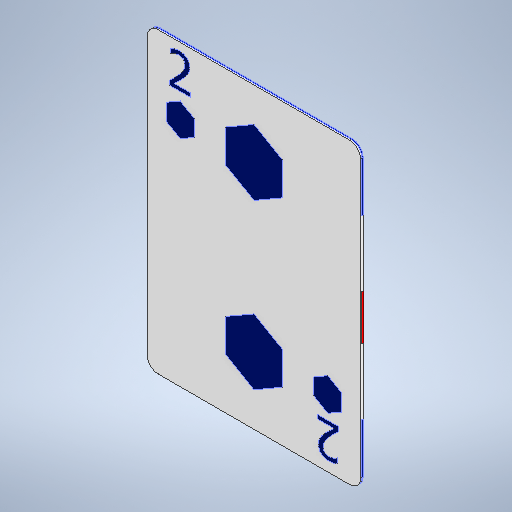
# Autodesk Inventor part: 2ofhexagons
Saved by Autodesk Inventor 2025 (Build 290162010, 162A)
## iProperties
Created: 2024-07-12
Part Number: 2ofhexagons
Material: Generic
Document SubType Name: Modeling
Designer: joshu
Density: 1 g/cm^3
Appearance: Default
Author: joshu
Autodesk Inventor part; units mm, degrees
(part 1 of 3)
ref_plane "YZ Plane" through (0, 0, 0) normal (1, 0, 0) x (0, 1, 0)
ref_plane "XZ Plane" through (0, 0, 0) normal (0, 1, 0) x (-1, 0, 0)
ref_plane "XY Plane" through (0, 0, 0) normal (0, 0, 1) x (1, 0, 0)
sketch "Sketch1" plane through (0, 0, 0) normal (0, 0, 1) x (1, 0, 0)
  line L0 (0, 0) -> (63.5, 0)
  line L1 (63.5, 0) -> (63.5, 88.9)
  line L2 (63.5, 88.9) -> (0, 88.9)
  line L3 (0, 88.9) -> (0, 0)
  line L4 (31.7966, 44.45) -> (43.5019, 51.0525)
  line L5 (43.5019, 51.0525) -> (43.5019, 65.3384)
  line L6 (43.5019, 65.3384) -> (31.75, 72.2052)
  line L7 (31.75, 72.2052) -> (19.9413, 65.5444)
  line L8 (19.9413, 65.5444) -> (19.9413, 51.51)
  line L9 (19.9413, 51.51) -> (31.7966, 44.45)
  line L10 (20.9808, 64.9373) -> (31.7409, 71.0066)
  line L11 (31.7409, 71.0066) -> (42.4624, 64.7418)
  line L12 (42.4624, 64.7418) -> (42.4624, 51.6596)
  line L13 (42.4624, 51.6596) -> (31.8107, 45.6515)
  line L14 (31.8107, 45.6515) -> (20.9808, 52.1009)
  line L15 (20.9808, 52.1009) -> (20.9808, 64.9373)
  line L16 (42.0481, 52.1761) -> (31.9218, 46.3281)
  line L17 (31.5408, 46.3613) -> (21.4951, 52.278)
  line L18 (38.5023, 66.4814) -> (31.9911, 66.4814)
  line L19 (38.6905, 66.1004) -> (38.6905, 61.5459)
  line L20 (38.3095, 62.9084) -> (37.0962, 62.9084)
  line L21 (37.0962, 62.9084) -> (37.0962, 62.5274)
  line L22 (37.0962, 62.5274) -> (38.3095, 62.5274)
  arc A0 (31.6066, 65.8741) -> (31.9876, 65.8741) centre (31.7971, 65.0383) ccw
  arc A1 (35.2141, 65.0547) -> (35.5951, 65.0547) centre (35.4046, 64.3169) ccw
  circle A2 centre (35.4046, 64.3169) radius 0.3175
  circle A3 centre (31.7971, 65.0383) radius 0.4127
  line L23 (41.2511, 61.3863) -> (41.2511, 54.1172)
  line L24 (40.8701, 59.3346) -> (39.5527, 59.3346)
  line L25 (39.4243, 58.9536) -> (40.8701, 58.9536)
  circle A4 centre (38.5, 60.6778) radius 0.508
  line L26 (39.4243, 58.9536) -> (38.6183, 59.7969)
  line L27 (39.5527, 59.3346) -> (38.9824, 59.9313)
  arc A5 (41.2511, 61.3863) -> (40.8701, 61.3863) centre (41.0606, 62.1232) ccw
  circle A6 centre (41.0606, 62.1232) radius 0.381
  line L28 (37.7054, 52.5185) -> (37.7054, 53.0908)
  circle A7 centre (37.8959, 53.9267) radius 0.4763
  line L29 (31.9911, 70.2625) -> (31.9911, 66.4814)
  line L30 (31.9876, 66.1004) -> (31.9876, 65.8741)
  line L31 (31.9876, 66.1004) -> (35.2141, 66.1004)
  line L32 (35.2141, 65.0547) -> (35.2141, 66.1004)
  line L33 (35.5951, 66.1004) -> (35.5951, 65.0547)
  line L34 (35.5951, 66.1004) -> (38.3095, 66.1004)
  line L35 (38.6905, 66.1004) -> (39.1584, 66.1004)
  line L36 (31.9876, 70.2646) -> (38.5023, 66.4814)
  line L37 (39.1584, 66.1004) -> (42.0481, 64.4224)
  line L38 (38.3095, 61.5459) -> (38.3095, 62.5274)
  line L39 (38.3095, 62.9084) -> (38.3095, 66.1004)
  arc A8 (38.3095, 61.5459) -> (38.6183, 59.7969) centre (38.5, 60.6778) ccw
  arc A9 (38.9824, 59.9313) -> (38.6905, 61.5459) centre (38.5, 60.6778) ccw
  line L40 (40.8701, 54.1172) -> (40.8701, 58.9536)
  line L41 (40.8701, 59.3346) -> (40.8701, 61.3863)
  line L42 (42.0481, 54.1172) -> (41.2511, 54.1172)
  line L43 (40.8701, 54.1172) -> (38.7317, 54.1172)
  line L44 (38.7282, 53.737) -> (42.0481, 53.737)
  line L45 (38.0845, 53.0941) -> (38.0845, 52.3272)
  arc A10 (38.7317, 54.1172) -> (37.7054, 53.0908) centre (37.8959, 53.9267) ccw
  arc A11 (38.0845, 53.0941) -> (38.7282, 53.737) centre (37.8959, 53.9267) ccw
  line L46 (42.0481, 64.4224) -> (42.0481, 54.1172)
  line L47 (42.0481, 53.737) -> (42.0481, 52.1761)
  line L48 (29.0948, 67.2715) -> (29.0948, 67.5351)
  line L49 (29.4758, 67.2715) -> (31.6066, 68.502)
  line L50 (29.0948, 67.5351) -> (31.6066, 68.9857)
  line L51 (31.6066, 65.8741) -> (31.6066, 68.502)
  line L52 (31.6066, 68.9857) -> (31.6066, 70.2564)
  line L53 (31.9218, 49.1234) -> (37.7054, 52.5185)
  line L54 (31.9218, 48.7095) -> (38.0845, 52.3272)
  line L55 (21.4951, 52.9132) -> (25.9629, 52.9132)
  line L56 (25.9629, 52.5322) -> (21.4951, 52.5322)
  line L57 (21.4951, 52.5322) -> (21.4951, 52.9132)
  line L58 (25.9629, 55.4481) -> (26.3439, 55.4481)
  line L59 (25.9629, 55.4481) -> (26.9185, 55.4481)
  line L60 (26.9185, 55.4481) -> (26.9185, 55.0671)
  line L61 (26.9185, 55.0671) -> (26.3439, 55.0671)
  line L62 (25.9629, 55.0671) -> (25.9629, 55.4481)
  line L63 (26.3439, 52.4415) -> (31.5408, 49.4741)
  line L64 (31.5408, 49.8815) -> (26.3439, 52.8489)
  arc A12 (31.9218, 51.0535) -> (31.5408, 51.0535) centre (31.7313, 51.824) ccw
  circle A13 centre (31.7313, 51.824) radius 0.4127
  arc A14 (25.9629, 51.8703) -> (26.3439, 51.8703) centre (26.1534, 51.0373) ccw
  circle A15 centre (26.1534, 51.0373) radius 0.4762
  line L65 (26.3439, 55.0671) -> (26.3439, 52.8489)
  line L66 (26.3439, 52.4415) -> (26.3439, 51.8703)
  line L67 (25.9629, 51.8703) -> (25.9629, 52.5322)
  line L68 (25.9629, 52.9132) -> (25.9629, 55.4481)
  line L69 (31.5408, 51.0535) -> (31.5408, 49.8815)
  line L70 (31.5408, 49.4741) -> (31.5408, 46.3613)
  line L71 (31.9218, 46.3613) -> (31.9218, 48.7095)
  line L72 (31.9218, 49.1234) -> (31.9218, 51.0535)
  line L73 (31.9218, 46.3613) -> (31.9218, 46.3281)
  arc A16 (29.0948, 64.6116) -> (29.4758, 64.6116) centre (29.2853, 63.9396) ccw
  circle A17 centre (29.2853, 63.9396) radius 0.3175
  line L74 (22.9961, 65.2838) -> (29.0948, 65.2838)
  line L75 (25.8093, 61.9378) -> (26.9185, 61.9378)
  line L76 (26.9185, 61.9378) -> (26.9185, 61.5568)
  line L77 (26.9185, 61.5568) -> (25.8093, 61.5568)
  line L78 (25.8093, 61.5568) -> (25.8093, 61.6173)
  line L79 (21.4951, 59.3346) -> (22.2343, 59.3346)
  line L80 (22.6153, 59.3346) -> (22.6153, 58.9536)
  line L81 (22.2343, 58.9536) -> (21.4951, 58.9536)
  line L82 (22.6153, 57.4638) -> (26.9185, 57.4638)
  line L83 (26.9185, 57.4638) -> (26.9185, 57.0828)
  line L84 (26.9185, 57.0828) -> (22.6153, 57.0828)
  line L85 (22.2343, 59.3346) -> (22.2343, 61.6532)
  line L86 (22.6153, 61.5038) -> (22.6153, 59.3346)
  line L87 (22.2343, 61.6532) -> (25.4283, 64.441)
  line L88 (22.6153, 61.5038) -> (25.4283, 63.959)
  arc A18 (25.4283, 60.5021) -> (25.8093, 60.5021) centre (25.6188, 59.7969) ccw
  circle A19 centre (25.6188, 59.7969) radius 0.3493
  line L89 (21.4951, 64.4169) -> (22.3363, 64.9028)
  line L90 (22.9961, 65.2838) -> (31.6066, 70.2564)
  line L91 (29.0948, 64.9028) -> (25.8093, 64.9028)
  line L92 (25.4283, 64.9028) -> (22.3363, 64.9028)
  line L93 (25.4283, 64.441) -> (25.4283, 64.9028)
  line L94 (29.4758, 64.6116) -> (29.4758, 67.2715)
  line L95 (25.8093, 64.9028) -> (25.8093, 61.9378)
  line L96 (25.8093, 61.5568) -> (25.8093, 60.5021)
  line L97 (25.4283, 60.075) -> (25.4283, 60.0896)
  line L98 (25.4283, 60.5021) -> (25.4283, 63.959)
  line L99 (21.4951, 52.278) -> (21.4951, 58.9536)
  line L100 (21.4951, 59.3346) -> (21.4951, 64.4169)
  line L101 (22.6153, 57.4638) -> (22.6153, 58.9536)
  line L102 (29.0948, 67.2715) -> (29.0948, 65.2838)
  line L103 (29.0948, 64.9028) -> (29.0948, 64.6116)
  line L104 (26.9185, 58.9484) -> (28.0615, 58.9484)
  line L105 (28.0615, 58.9484) -> (28.0615, 61.2883)
  line L106 (28.0615, 63.1194) -> (26.9185, 63.1194)
  line L107 (26.9185, 63.1194) -> (26.9185, 58.9484)
  line L108 (29.8151, 63.1194) -> (30.9581, 63.1194)
  line L109 (30.9581, 63.1194) -> (30.9581, 58.9484)
  line L110 (30.9581, 58.9484) -> (29.8151, 58.9484)
  line L111 (29.8151, 60.7795) -> (29.8151, 63.1194)
  line L112 (29.8151, 58.9484) -> (28.0615, 61.2883)
  line L113 (28.0615, 63.1194) -> (29.8151, 60.7795)
  line L114 (31.4657, 63.1194) -> (32.6087, 63.1194)
  line L115 (32.6087, 58.9484) -> (31.4657, 58.9484)
  line L116 (31.4657, 58.9484) -> (31.4657, 63.1194)
  line L117 (31.4657, 63.1194) -> (33.8556, 63.1194)
  line L118 (33.8556, 63.1194) -> (33.8556, 61.9764)
  line L119 (33.8556, 61.9764) -> (32.6087, 61.9764)
  line L120 (31.4657, 61.9764) -> (31.4657, 63.1194)
  line L121 (32.6087, 61.5255) -> (33.8556, 61.5255)
  line L122 (33.8556, 61.5255) -> (33.8556, 60.5095)
  line L123 (33.8556, 60.5095) -> (32.6087, 60.5095)
  line L124 (31.4657, 60.5095) -> (31.4657, 61.5255)
  line L125 (31.4657, 58.9484) -> (33.8556, 58.9484)
  line L126 (33.8556, 58.9484) -> (33.8556, 60.0914)
  line L127 (33.8556, 60.0914) -> (32.6087, 60.0914)
  line L128 (31.4657, 60.0914) -> (31.4657, 58.9484)
  line L129 (32.6087, 61.9764) -> (32.6087, 61.5255)
  line L130 (32.6087, 60.5095) -> (32.6087, 60.0914)
  line L131 (37.0962, 63.1114) -> (34.2865, 63.1114)
  line L132 (34.2865, 63.1114) -> (34.2865, 62.0954)
  line L133 (37.0962, 62.0954) -> (37.0962, 63.1114)
  line L134 (36.261, 62.0954) -> (36.261, 58.9484)
  line L135 (36.261, 58.9484) -> (35.118, 58.9484)
  line L136 (35.118, 58.9484) -> (35.118, 62.0954)
  line L137 (35.118, 62.0954) -> (35.2141, 62.0954)
  line L138 (34.2865, 62.0954) -> (35.118, 62.0954)
  line L139 (36.261, 62.0954) -> (37.0962, 62.0954)
  line L140 (26.9185, 57.9141) -> (28.0615, 57.9141)
  line L141 (28.0615, 57.9141) -> (28.0615, 54.753)
  line L142 (28.0615, 53.737) -> (26.9185, 53.737)
  line L143 (26.9185, 53.737) -> (26.9185, 57.9141)
  line L144 (26.9185, 53.737) -> (29.1789, 53.737)
  line L145 (29.1789, 53.737) -> (29.1789, 54.753)
  line L146 (29.1789, 54.753) -> (28.0615, 54.753)
  line L147 (26.9185, 54.753) -> (26.9185, 53.737)
  line L148 (29.3943, 53.737) -> (30.5373, 53.737)
  line L149 (30.5373, 53.737) -> (30.8468, 54.4929)
  line L150 (30.8468, 54.4929) -> (32.1168, 54.4929)
  line L151 (30.8468, 57.9141) -> (32.1168, 57.9141)
  line L152 (29.3943, 53.737) -> (30.8468, 57.9141)
  line L153 (32.4486, 53.737) -> (33.5916, 53.737)
  line L154 (32.4486, 53.737) -> (32.1168, 54.4929)
  line L155 (33.5916, 53.737) -> (32.1168, 57.9141)
  line L156 (31.0435, 55.3657) -> (31.9218, 55.3657)
  line L157 (31.9218, 55.3657) -> (31.4818, 56.4223)
  line L158 (31.4818, 56.4223) -> (31.0435, 55.3657)
  line L159 (33.911, 53.737) -> (33.911, 57.9141)
  line L160 (33.911, 57.9141) -> (35.876, 57.9141)
  line L161 (33.911, 53.737) -> (35.876, 53.737)
  line L162 (35.0032, 54.6929) -> (35.0032, 55.4427)
  line L163 (35.0032, 56.2657) -> (35.0032, 56.9462)
  line L164 (35.0032, 56.9462) -> (35.4388, 56.9462)
  line L165 (35.0032, 56.2657) -> (35.4388, 56.2657)
  arc A20 (35.4388, 56.2657) -> (35.4388, 56.9462) centre (35.3333, 56.606) ccw
  line L166 (35.0032, 55.4427) -> (35.5978, 55.4427)
  line L167 (35.0032, 54.6929) -> (35.5896, 54.6929)
  arc A21 (35.5896, 54.6929) -> (35.5978, 55.4427) centre (35.5605, 55.0681) ccw
  arc A22 (36.3387, 56.0044) -> (35.876, 57.9141) centre (35.6477, 56.8479) ccw
  arc A23 (35.876, 53.737) -> (36.3387, 56.0044) centre (35.9369, 54.9055) ccw
  arc A24 (22.2343, 54.7316) -> (22.6153, 54.7316) centre (22.4248, 54.0266) ccw
  circle A25 centre (22.4248, 54.0266) radius 0.3493
  line L168 (22.2343, 58.9536) -> (22.2343, 54.7316)
  line L169 (22.6153, 54.7316) -> (22.6153, 57.0828)
  line L170 (31.9911, 70.2625) -> (38.5023, 66.4814)
  line L171 (31.9911, 66.4814) -> (38.5023, 66.4814)
  line L172 (31.9911, 66.4814) -> (31.9911, 70.2625)
  line L173 (22.2842, 29.8053) -> (21.5449, 29.8027)
  line L174 (22.6665, 29.4256) -> (22.6651, 29.8066)
  line L175 (22.6601, 31.2964) -> (22.6651, 29.8066)
  line L176 (21.5462, 29.4217) -> (22.2855, 29.4243)
  line L177 (21.523, 36.2241) -> (21.5243, 35.8431)
  line L178 (21.5221, 36.4783) -> (21.5449, 29.8027)
  line L179 (21.5243, 35.8431) -> (25.9921, 35.8584)
  line L180 (25.9908, 36.2394) -> (21.523, 36.2241)
  line L181 (22.6507, 34.0285) -> (22.6587, 31.6774)
  line L182 (22.2842, 29.8053) -> (22.2697, 34.0272)
  circle A26 centre (22.4578, 34.7329) radius 0.3493
  arc A27 (22.6507, 34.0285) -> (22.2697, 34.0272) centre (22.4578, 34.7329) ccw
  line L183 (39.2326, 22.7164) -> (42.1166, 24.4043)
  line L184 (38.7647, 22.7148) -> (39.2326, 22.7164)
  line L185 (38.3728, 25.9055) -> (38.3837, 22.7135)
  line L186 (38.7647, 22.7148) -> (38.7491, 27.2693)
  line L187 (38.3728, 25.9055) -> (37.1595, 25.9014)
  line L188 (37.1582, 26.2824) -> (38.3715, 26.2865)
  line L189 (35.6693, 22.7042) -> (38.3837, 22.7135)
  line L190 (35.2848, 23.7486) -> (35.2883, 22.7029)
  circle A28 centre (38.5556, 28.1368) radius 0.508
  circle A29 centre (35.4727, 24.4871) radius 0.3175
  arc A30 (35.6658, 23.7499) -> (35.2848, 23.7486) centre (35.4727, 24.4871) ccw
  line L191 (32.0618, 22.6919) -> (35.2883, 22.7029)
  arc A31 (32.0611, 22.9182) -> (31.6801, 22.9169) centre (31.8677, 23.7534) ccw
  line L192 (35.6693, 22.7042) -> (35.6658, 23.7499)
  line L193 (22.6601, 31.2964) -> (26.9632, 31.3111)
  line L194 (26.9619, 31.6921) -> (22.6587, 31.6774)
  line L195 (26.9632, 31.3111) -> (26.9619, 31.6921)
  circle A32 centre (26.1761, 37.735) radius 0.4762
  arc A33 (26.3695, 36.9026) -> (25.9885, 36.9013) centre (26.1761, 37.735) ccw
  line L196 (26.3714, 36.3314) -> (26.3695, 36.9026)
  line L197 (25.9885, 36.9013) -> (25.9908, 36.2394)
  line L198 (26.9563, 33.3268) -> (26.955, 33.7078)
  line L199 (26.3804, 33.7058) -> (26.3728, 35.924)
  line L200 (26.955, 33.7078) -> (26.3804, 33.7058)
  line L201 (25.9921, 35.8584) -> (26.0007, 33.3235)
  line L202 (25.9994, 33.7045) -> (26.0007, 33.3235)
  line L203 (26.0007, 33.3235) -> (26.3817, 33.3248)
  line L204 (26.0007, 33.3235) -> (26.9563, 33.3268)
  line L205 (30.5693, 35.0503) -> (30.8814, 34.2954)
  line L206 (29.2143, 34.0297) -> (28.097, 34.0258)
  line L207 (29.4263, 35.0464) -> (30.5693, 35.0503)
  line L208 (26.954, 34.0219) -> (26.9505, 35.0379)
  line L209 (29.4263, 35.0464) -> (30.8931, 30.8743)
  line L210 (22.2934, 27.1057) -> (25.4969, 24.3288)
  line L211 (22.6739, 27.2564) -> (25.4952, 24.8108)
  line L212 (25.868, 27.2143) -> (25.8644, 28.2691)
  line L213 (25.4819, 28.6948) -> (25.482, 28.6802)
  line L214 (25.4834, 28.2678) -> (25.4952, 24.8108)
  line L215 (25.8795, 23.8684) -> (25.8693, 26.8333)
  line L216 (25.4969, 24.3288) -> (25.4985, 23.8671)
  line L217 (25.4985, 23.8671) -> (22.4066, 23.8565)
  line L218 (21.5462, 29.4217) -> (21.5636, 24.3395)
  line L219 (21.5636, 24.3395) -> (22.4066, 23.8565)
  circle A34 centre (25.6715, 28.9736) radius 0.3493
  line L220 (31.081, 33.4233) -> (31.9594, 33.4263)
  line L221 (31.523, 32.3682) -> (31.081, 33.4233)
  line L222 (31.9594, 33.4263) -> (31.523, 32.3682)
  line L223 (30.8814, 34.2954) -> (32.1514, 34.2998)
  line L224 (29.2108, 35.0457) -> (29.2143, 34.0297)
  line L225 (28.1078, 30.8647) -> (28.097, 34.0258)
  line L226 (28.0935, 35.0418) -> (26.9505, 35.0379)
  line L227 (26.9505, 35.0379) -> (26.9648, 30.8608)
  line L228 (26.9505, 35.0379) -> (29.2108, 35.0457)
  line L229 (26.9648, 30.8608) -> (28.1078, 30.8647)
  line L230 (30.8931, 30.8743) -> (32.1631, 30.8786)
  line L231 (32.4805, 35.0569) -> (32.1514, 34.2998)
  line L232 (28.1256, 25.6594) -> (26.9826, 25.6555)
  line L233 (25.8693, 26.8333) -> (26.9785, 26.8371)
  line L234 (26.9772, 27.2181) -> (25.868, 27.2143)
  line L235 (25.868, 27.2143) -> (25.8682, 27.1538)
  line L236 (26.9785, 26.8371) -> (26.9772, 27.2181)
  line L237 (22.2855, 29.4243) -> (22.2934, 27.1057)
  line L238 (22.6739, 27.2564) -> (22.6665, 29.4256)
  arc A35 (25.8644, 28.2691) -> (25.4834, 28.2678) centre (25.6715, 28.9736) ccw
  line L239 (26.9826, 25.6555) -> (26.9683, 29.8265)
  line L240 (26.9683, 29.8265) -> (28.1113, 29.8304)
  line L241 (31.0079, 29.8403) -> (29.8649, 29.8364)
  line L242 (32.6585, 29.846) -> (31.5155, 29.8421)
  line L243 (32.6673, 27.2689) -> (33.9142, 27.2732)
  line L244 (31.5155, 29.8421) -> (33.9054, 29.8503)
  line L245 (33.9054, 29.8503) -> (33.9093, 28.7073)
  line L246 (33.9093, 28.7073) -> (32.6624, 28.703)
  line L247 (31.5194, 28.6991) -> (31.5155, 29.8421)
  line L248 (32.6638, 28.2849) -> (32.6624, 28.703)
  line L249 (33.9107, 28.2892) -> (32.6638, 28.2849)
  line L250 (33.9142, 27.2732) -> (33.9107, 28.2892)
  line L251 (31.5208, 28.281) -> (31.5243, 27.265)
  line L252 (32.6688, 26.818) -> (32.6673, 27.2689)
  line L253 (35.0461, 31.8563) -> (35.4817, 31.8578)
  line L254 (35.0384, 34.1097) -> (35.6249, 34.1117)
  line L255 (35.041, 33.3599) -> (35.6356, 33.3619)
  line L256 (33.9429, 35.0619) -> (35.9079, 35.0686)
  line L257 (31.5582, 39.3166) -> (31.5476, 42.4293)
  line L258 (31.9286, 42.4307) -> (31.9366, 40.0825)
  line L259 (31.9286, 42.4307) -> (31.9285, 42.4639)
  line L260 (35.0438, 32.5368) -> (35.0461, 31.8563)
  line L261 (33.9572, 30.8847) -> (35.9222, 30.8915)
  line L262 (33.6235, 35.0608) -> (32.1631, 30.8786)
  line L263 (32.4805, 35.0569) -> (33.6235, 35.0608)
  line L264 (35.0438, 32.5368) -> (35.4794, 32.5383)
  line L265 (33.9429, 35.0619) -> (33.9572, 30.8847)
  arc A36 (35.4817, 31.8578) -> (35.4794, 32.5383) centre (35.375, 32.1977) ccw
  line L266 (35.0384, 34.1097) -> (35.041, 33.3599)
  arc A37 (35.6356, 33.3619) -> (35.6249, 34.1117) centre (35.597, 33.7363) ccw
  arc A38 (35.9222, 30.8915) -> (36.3784, 32.8027) centre (35.6902, 31.9569) ccw
  arc A39 (36.3784, 32.8027) -> (35.9079, 35.0686) centre (35.9728, 33.9003) ccw
  line L267 (37.1595, 25.9014) -> (37.1582, 26.2824)
  line L268 (36.3108, 29.8585) -> (35.1678, 29.8546)
  line L269 (34.347, 26.7047) -> (35.1786, 26.7075)
  line L270 (35.1678, 29.8546) -> (35.1786, 26.7075)
  line L271 (35.1786, 26.7075) -> (35.2746, 26.7079)
  line L272 (36.3215, 26.7115) -> (36.3108, 29.8585)
  line L273 (36.3215, 26.7115) -> (37.1567, 26.7143)
  line L274 (34.3505, 25.6887) -> (34.347, 26.7047)
  line L275 (37.1602, 25.6983) -> (34.3505, 25.6887)
  line L276 (37.1567, 26.7143) -> (37.1602, 25.6983)
  line L277 (31.7966, 44.45) -> (43.6866, 37.5937)
  line L278 (42.5183, 36.9086) -> (31.7603, 43.0725)
  line L279 (42.0747, 36.6505) -> (31.9285, 42.4639)
  line L280 (31.938, 39.6686) -> (37.7332, 36.2932)
  line L281 (31.9366, 40.0825) -> (38.1116, 36.4859)
  line L282 (31.938, 39.6686) -> (31.9446, 37.7385)
  line L283 (29.1731, 21.5109) -> (29.174, 21.2473)
  line L284 (29.5541, 21.5122) -> (31.6891, 20.289)
  line L285 (29.174, 21.2473) -> (31.6907, 19.8053)
  line L286 (31.6801, 22.9169) -> (31.6891, 20.289)
  line L287 (31.6907, 19.8053) -> (31.6951, 18.5346)
  circle A40 centre (29.3522, 24.8434) radius 0.3175
  arc A41 (29.545, 24.1721) -> (29.164, 24.1708) centre (29.3522, 24.8434) ccw
  line L288 (29.165, 23.8796) -> (29.164, 24.1708)
  line L289 (29.165, 23.8796) -> (25.8795, 23.8684)
  line L290 (23.0676, 23.4777) -> (29.1663, 23.4986)
  line L291 (29.545, 24.1721) -> (29.5541, 21.5122)
  line L292 (29.1731, 21.5109) -> (29.1663, 23.4986)
  line L293 (23.0676, 23.4777) -> (31.6951, 18.5346)
  line L294 (32.0618, 22.6919) -> (32.0611, 22.9182)
  line L295 (32.0796, 18.5298) -> (32.0667, 22.3109)
  line L296 (21.12, 24.0813) -> (31.8964, 17.907)
  circle A42 centre (31.8677, 23.7534) radius 0.4127
  line L297 (31.8713, 16.6404) -> (19.9676, 23.5047)
  line L298 (21.0767, 36.7309) -> (21.12, 24.0813)
  line L299 (19.9676, 23.5047) -> (19.9586, 37.4674)
  circle A43 centre (31.7568, 36.9673) radius 0.4127
  line L300 (31.5476, 42.4293) -> (21.5221, 36.4783)
  line L301 (19.9586, 37.4674) -> (31.7966, 44.45)
  line L302 (31.7603, 43.0725) -> (21.0767, 36.7309)
  line L303 (31.5596, 38.9092) -> (26.3728, 35.924)
  line L304 (26.3714, 36.3314) -> (31.5582, 39.3166)
  line L305 (31.5636, 37.7372) -> (31.5596, 38.9092)
  arc A44 (31.5636, 37.7372) -> (31.9446, 37.7385) centre (31.7568, 36.9673) ccw
  circle A45 centre (41.1212, 26.7001) radius 0.381
  line L306 (40.9212, 29.488) -> (39.6037, 29.4835)
  line L307 (39.474, 29.8641) -> (40.9199, 29.869)
  line L308 (37.7332, 36.2932) -> (37.7351, 35.7209)
  circle A46 centre (37.9285, 34.8858) radius 0.4763
  line L309 (38.7601, 35.0783) -> (42.08, 35.0897)
  line L310 (38.1142, 35.719) -> (38.1116, 36.4859)
  arc A47 (37.7351, 35.7209) -> (38.7649, 34.6981) centre (37.9285, 34.8858) ccw
  arc A48 (38.7601, 35.0783) -> (38.1142, 35.719) centre (37.9285, 34.8858) ccw
  line L311 (42.08, 35.0897) -> (42.0747, 36.6505)
  line L312 (43.6866, 37.5937) -> (43.6957, 23.5059)
  line L313 (42.562, 24.1393) -> (42.5183, 36.9086)
  line L314 (41.3092, 27.4376) -> (41.2843, 34.7068)
  line L315 (39.474, 29.8641) -> (38.6709, 29.0181)
  line L316 (39.6037, 29.4835) -> (39.0355, 28.8849)
  arc A49 (40.9282, 27.4363) -> (41.3092, 27.4376) centre (41.1212, 26.7001) ccw
  line L317 (38.3681, 27.268) -> (38.3715, 26.2865)
  arc A50 (38.7491, 27.2693) -> (39.0355, 28.8849) centre (38.5556, 28.1368) ccw
  line L318 (40.9212, 29.488) -> (40.9282, 27.4363)
  line L319 (42.1166, 24.4043) -> (42.0813, 34.7095)
  line L320 (42.0813, 34.7095) -> (41.2843, 34.7068)
  line L321 (40.9033, 34.7055) -> (40.9199, 29.869)
  line L322 (40.9033, 34.7055) -> (38.7649, 34.6981)
  arc A51 (38.6709, 29.0181) -> (38.3681, 27.268) centre (38.5556, 28.1368) ccw
  line L323 (43.6957, 23.5059) -> (31.8713, 16.6404)
  line L324 (31.8964, 17.907) -> (42.562, 24.1393)
  line L325 (38.5779, 22.3332) -> (32.0667, 22.3109)
  line L326 (32.0761, 18.5277) -> (38.5779, 22.3332)
  line L327 (32.0667, 22.3109) -> (32.0796, 18.5298)
  line L328 (32.0796, 18.5298) -> (38.5779, 22.3332)
  line L329 (32.0667, 22.3109) -> (38.5779, 22.3332)
  line L330 (28.1113, 29.8304) -> (28.1193, 27.4905)
  line L331 (29.8792, 25.6654) -> (31.0222, 25.6693)
  line L332 (31.0222, 25.6693) -> (31.0079, 29.8403)
  line L333 (29.8649, 29.8364) -> (28.1193, 27.4905)
  line L334 (33.9158, 26.8222) -> (32.6688, 26.818)
  line L335 (31.5298, 25.6711) -> (33.9197, 25.6792)
  line L336 (33.9197, 25.6792) -> (33.9158, 26.8222)
  line L337 (31.5155, 29.8421) -> (31.5298, 25.6711)
  line L338 (31.5298, 25.6711) -> (32.6728, 25.675)
  line L339 (29.8712, 28.0053) -> (29.8792, 25.6654)
  line L340 (28.1256, 25.6594) -> (29.8712, 28.0053)
  line L341 (31.5258, 26.8141) -> (31.5298, 25.6711)
  line L342 (31.75, 80.4139) -> (44.6823, 72.8573)
  line L343 (44.6823, 72.8573) -> (54.0323, 76.3351)
  line L344 (54.0323, 76.3351) -> (63.5, 70.8029)
  line L345 (31.75, 72.2052) -> (31.75, 88.9) construction
  line L346 (31.75, 80.4139) -> (18.8177, 72.8573)
  line L347 (18.8177, 72.8573) -> (9.4677, 76.3351)
  line L348 (9.4677, 76.3351) -> (0, 70.8029)
  line L349 (29.1432, 44.45) -> (63.5, 44.45) construction
  line L350 (31.75, 8.4861) -> (44.6823, 16.0427)
  line L351 (44.6823, 16.0427) -> (54.0323, 12.5649)
  line L352 (31.75, 8.4861) -> (18.8177, 16.0427)
  line L353 (18.8177, 16.0427) -> (9.4677, 12.5649)
  line L354 (9.4677, 12.5649) -> (0, 18.0971)
  line L355 (54.0323, 12.5649) -> (63.5, 18.0971)
  line L356 (0, 51.1737) -> (17.8526, 51.1737)
  line L357 (17.8526, 51.1737) -> (29.1432, 44.45)
  line L358 (0, 37.7263) -> (17.8526, 37.7263)
  line L359 (17.8526, 37.7263) -> (29.1432, 44.45)
  line L360 (63.5, 51.1737) -> (45.6474, 51.1737)
  line L361 (45.6474, 51.1737) -> (34.3568, 44.45)
  line L362 (45.6474, 37.7263) -> (34.3568, 44.45)
  line L363 (63.5, 37.7263) -> (45.6474, 37.7263)
  point P0 (31.7785, 58.3278)
  point P1 (31.8262, 30.4638)
  dimension "d0" = 63.5
  dimension "d1" = 88.9
  constraints: 728 end point, 89 parallel, 64 point on circle, 50 centre point, 37 horizontal, 22 point on line, 21 perpendicular, 20 coincident, 17 symmetric about line, 5 vertical, 4 collinear, 2 midpoint, 11 other
  measures "d0" distance of L2.end L1.end
  measures "d1" distance of L1.end L0.end
extrude "Extrusion1" add sketch "Sketch1" along normal blind 0.4 contours L3 L354 L353 L352 L350 L351 L355 L1 L0 | L3 L2 L1 L344 L343 L342 L346 L347 L348 | L9 L8 L7 L6 L5 L4 | L277 L312 L323 L297 L299 L301 | L16 L73 L71 L54 L45 A11 L44 L47 | L17 L99 L56 L67 A14 L66 L63 L70 | L18 L29 L36 | L35 L37 L46 L42 L23 A5 L41 L24 L27 A9 L19 | L20 L133 L131 L132 L138 L136 L135 L134 L139 L22 L38 A8 L26 L25 L40 L43 A10 L28 L53 L72 A12 L69 L64 L65 L61 L143 L142 L144 L145 L146 L141 L140 L82 L101 L80 L86 L88 L98 A18 L96 L77 L107 L104 L105 L112 L110 L109 L108 L111 L113 L106 L75 L95 L91 L103 A16 L94 L49 L51 A0 L30 L31 L32 A1 L33 L34 L39 | L59 L58 L62 L68 L55 L99 L81 L168 A24 L169 L84 L143 | A2 | A3 | A4 | A6 | A7 | L102 L74 L90 L52 L50 L48 | A13 | A15 | A17 | L100 L89 L92 L93 L87 L85 L79 | A19 | L158 L157 L156 | L162 L166 A21 L167 | L163 L164 A20 L165 | A25 | L173 L178 L179 L201 L203 L204 L227 L194 L181 A27 L182 | L227 L229 L225 L206 L224 L228 L226 L208 L200 L199 L303 L305 A44 L282 L280 L308 A47 L322 L321 L307 L315 A51 L317 L188 L276 L273 L272 L268 L270 L269 L274 L275 L187 L185 L189 L192 A30 L190 L191 L294 A31 L286 L284 L291 A41 L288 L289 L215 L233 L239 L232 L340 L339 L331 L332 L241 L333 L330 L240 L234 L212 A35 L214 L211 L238 L174 L175 L193 | L176 L237 L210 L216 L217 L219 L218 | L300 L257 L304 L196 A33 L197 L180 L178 | A26 | L184 L186 A50 L316 L306 L318 A49 L314 L320 L319 L183 | A28 | A29 | A32 | A34 | L220 L222 L221 | L260 L264 A36 L253 | L254 A37 L255 L266 | L259 L279 L311 L309 A48 L310 L281 L258 | L283 L285 L287 L293 L290 L292 | A40 | L295 L325 L326 | A42 | A43 | A45 | A46
sketch "Sketch3" plane through (0, 0, 0.4) normal (0, 0, 1) x (1, 0, 0)
  line L0 (0, 0) -> (63.5, 0)
  line L1 (63.5, 0) -> (63.5, 88.9)
  line L2 (63.5, 88.9) -> (0, 88.9)
  line L3 (0, 88.9) -> (0, 0)
  line L4 (22.2343, 58.9536) -> (21.4951, 58.9536)
  line L5 (22.6153, 59.3346) -> (22.6153, 58.9536)
  line L6 (22.6153, 57.4638) -> (22.6153, 58.9536)
  line L7 (21.4951, 59.3346) -> (22.2343, 59.3346)
  line L8 (21.4951, 52.5322) -> (21.4951, 52.9132)
  line L9 (21.4951, 52.278) -> (21.4951, 58.9536)
  line L10 (21.4951, 52.9132) -> (25.9629, 52.9132)
  line L11 (25.9629, 52.5322) -> (21.4951, 52.5322)
  line L12 (22.6153, 54.7316) -> (22.6153, 57.0828)
  line L13 (22.2343, 58.9536) -> (22.2343, 54.7316)
  circle A0 centre (22.4248, 54.0266) radius 0.3493
  arc A1 (22.2343, 54.7316) -> (22.6153, 54.7316) centre (22.4248, 54.0266) ccw
  line L14 (39.1584, 66.1004) -> (42.0481, 64.4224)
  line L15 (38.6905, 66.1004) -> (39.1584, 66.1004)
  line L16 (38.3095, 62.9084) -> (38.3095, 66.1004)
  line L17 (38.6905, 66.1004) -> (38.6905, 61.5459)
  line L18 (38.3095, 62.9084) -> (37.0962, 62.9084)
  line L19 (37.0962, 62.5274) -> (38.3095, 62.5274)
  line L20 (35.5951, 66.1004) -> (38.3095, 66.1004)
  line L21 (35.2141, 65.0547) -> (35.2141, 66.1004)
  circle A2 centre (38.5, 60.6778) radius 0.508
  circle A3 centre (35.4046, 64.3169) radius 0.3175
  arc A4 (35.2141, 65.0547) -> (35.5951, 65.0547) centre (35.4046, 64.3169) ccw
  line L22 (31.9876, 66.1004) -> (35.2141, 66.1004)
  arc A5 (31.6066, 65.8741) -> (31.9876, 65.8741) centre (31.7971, 65.0383) ccw
  line L23 (35.5951, 66.1004) -> (35.5951, 65.0547)
  line L24 (22.6153, 57.4638) -> (26.9185, 57.4638)
  line L25 (26.9185, 57.0828) -> (22.6153, 57.0828)
  line L26 (26.9185, 57.4638) -> (26.9185, 57.0828)
  circle A6 centre (26.1534, 51.0373) radius 0.4762
  arc A7 (25.9629, 51.8703) -> (26.3439, 51.8703) centre (26.1534, 51.0373) ccw
  line L27 (26.3439, 52.4415) -> (26.3439, 51.8703)
  line L28 (25.9629, 51.8703) -> (25.9629, 52.5322)
  line L29 (26.9185, 55.4481) -> (26.9185, 55.0671)
  line L30 (26.3439, 55.0671) -> (26.3439, 52.8489)
  line L31 (26.9185, 55.0671) -> (26.3439, 55.0671)
  line L32 (25.9629, 52.9132) -> (25.9629, 55.4481)
  line L33 (25.9629, 55.0671) -> (25.9629, 55.4481)
  line L34 (25.9629, 55.4481) -> (26.3439, 55.4481)
  line L35 (25.9629, 55.4481) -> (26.9185, 55.4481)
  line L36 (30.5373, 53.737) -> (30.8468, 54.4929)
  line L37 (29.1789, 54.753) -> (28.0615, 54.753)
  line L38 (29.3943, 53.737) -> (30.5373, 53.737)
  line L39 (26.9185, 54.753) -> (26.9185, 53.737)
  line L40 (29.3943, 53.737) -> (30.8468, 57.9141)
  line L41 (22.2343, 61.6532) -> (25.4283, 64.441)
  line L42 (22.6153, 61.5038) -> (25.4283, 63.959)
  line L43 (25.8093, 61.5568) -> (25.8093, 60.5021)
  line L44 (25.4283, 60.075) -> (25.4283, 60.0896)
  line L45 (25.4283, 60.5021) -> (25.4283, 63.959)
  line L46 (25.8093, 64.9028) -> (25.8093, 61.9378)
  line L47 (25.4283, 64.441) -> (25.4283, 64.9028)
  line L48 (25.4283, 64.9028) -> (22.3363, 64.9028)
  line L49 (21.4951, 59.3346) -> (21.4951, 64.4169)
  line L50 (21.4951, 64.4169) -> (22.3363, 64.9028)
  circle A8 centre (25.6188, 59.7969) radius 0.3493
  line L51 (31.0435, 55.3657) -> (31.9218, 55.3657)
  line L52 (31.4818, 56.4223) -> (31.0435, 55.3657)
  line L53 (31.9218, 55.3657) -> (31.4818, 56.4223)
  line L54 (30.8468, 54.4929) -> (32.1168, 54.4929)
  line L55 (29.1789, 53.737) -> (29.1789, 54.753)
  line L56 (28.0615, 57.9141) -> (28.0615, 54.753)
  line L57 (28.0615, 53.737) -> (26.9185, 53.737)
  line L58 (26.9185, 53.737) -> (26.9185, 57.9141)
  line L59 (26.9185, 53.737) -> (29.1789, 53.737)
  line L60 (26.9185, 57.9141) -> (28.0615, 57.9141)
  line L61 (30.8468, 57.9141) -> (32.1168, 57.9141)
  line L62 (32.4486, 53.737) -> (32.1168, 54.4929)
  line L63 (28.0615, 63.1194) -> (26.9185, 63.1194)
  line L64 (25.8093, 61.9378) -> (26.9185, 61.9378)
  line L65 (26.9185, 61.5568) -> (25.8093, 61.5568)
  line L66 (25.8093, 61.5568) -> (25.8093, 61.6173)
  line L67 (26.9185, 61.9378) -> (26.9185, 61.5568)
  line L68 (22.2343, 59.3346) -> (22.2343, 61.6532)
  line L69 (22.6153, 61.5038) -> (22.6153, 59.3346)
  arc A9 (25.4283, 60.5021) -> (25.8093, 60.5021) centre (25.6188, 59.7969) ccw
  line L70 (26.9185, 63.1194) -> (26.9185, 58.9484)
  line L71 (26.9185, 58.9484) -> (28.0615, 58.9484)
  line L72 (30.9581, 58.9484) -> (29.8151, 58.9484)
  line L73 (32.6087, 58.9484) -> (31.4657, 58.9484)
  line L74 (32.6087, 61.5255) -> (33.8556, 61.5255)
  line L75 (31.4657, 58.9484) -> (33.8556, 58.9484)
  line L76 (33.8556, 58.9484) -> (33.8556, 60.0914)
  line L77 (33.8556, 60.0914) -> (32.6087, 60.0914)
  line L78 (31.4657, 60.0914) -> (31.4657, 58.9484)
  line L79 (32.6087, 60.5095) -> (32.6087, 60.0914)
  line L80 (33.8556, 60.5095) -> (32.6087, 60.5095)
  line L81 (33.8556, 61.5255) -> (33.8556, 60.5095)
  line L82 (31.4657, 60.5095) -> (31.4657, 61.5255)
  line L83 (32.6087, 61.9764) -> (32.6087, 61.5255)
  line L84 (35.0032, 56.9462) -> (35.4388, 56.9462)
  line L85 (35.0032, 54.6929) -> (35.5896, 54.6929)
  line L86 (35.0032, 55.4427) -> (35.5978, 55.4427)
  line L87 (33.911, 53.737) -> (35.876, 53.737)
  line L88 (31.5408, 49.4741) -> (31.5408, 46.3613)
  line L89 (31.9218, 46.3613) -> (31.9218, 48.7095)
  line L90 (31.9218, 46.3613) -> (31.9218, 46.3281)
  line L91 (35.0032, 56.2657) -> (35.0032, 56.9462)
  line L92 (33.911, 57.9141) -> (35.876, 57.9141)
  line L93 (33.5916, 53.737) -> (32.1168, 57.9141)
  line L94 (32.4486, 53.737) -> (33.5916, 53.737)
  line L95 (35.0032, 56.2657) -> (35.4388, 56.2657)
  line L96 (33.911, 53.737) -> (33.911, 57.9141)
  arc A10 (35.4388, 56.2657) -> (35.4388, 56.9462) centre (35.3333, 56.606) ccw
  line L97 (35.0032, 54.6929) -> (35.0032, 55.4427)
  arc A11 (35.5896, 54.6929) -> (35.5978, 55.4427) centre (35.5605, 55.0681) ccw
  arc A12 (36.3387, 56.0044) -> (35.876, 57.9141) centre (35.6477, 56.8479) ccw
  arc A13 (35.876, 53.737) -> (36.3387, 56.0044) centre (35.9369, 54.9055) ccw
  line L98 (37.0962, 62.9084) -> (37.0962, 62.5274)
  line L99 (36.261, 58.9484) -> (35.118, 58.9484)
  line L100 (34.2865, 62.0954) -> (35.118, 62.0954)
  line L101 (35.118, 58.9484) -> (35.118, 62.0954)
  line L102 (35.118, 62.0954) -> (35.2141, 62.0954)
  line L103 (36.261, 62.0954) -> (36.261, 58.9484)
  line L104 (36.261, 62.0954) -> (37.0962, 62.0954)
  line L105 (34.2865, 63.1114) -> (34.2865, 62.0954)
  line L106 (37.0962, 63.1114) -> (34.2865, 63.1114)
  line L107 (37.0962, 62.0954) -> (37.0962, 63.1114)
  line L108 (31.7966, 44.45) -> (43.5019, 51.0525)
  line L109 (42.4624, 51.6596) -> (31.8107, 45.6515)
  line L110 (42.0481, 52.1761) -> (31.9218, 46.3281)
  line L111 (31.9218, 49.1234) -> (37.7054, 52.5185)
  line L112 (31.9218, 48.7095) -> (38.0845, 52.3272)
  line L113 (31.9218, 49.1234) -> (31.9218, 51.0535)
  line L114 (29.0948, 67.2715) -> (29.0948, 67.5351)
  line L115 (29.4758, 67.2715) -> (31.6066, 68.502)
  line L116 (29.0948, 67.5351) -> (31.6066, 68.9857)
  line L117 (31.6066, 65.8741) -> (31.6066, 68.502)
  line L118 (31.6066, 68.9857) -> (31.6066, 70.2564)
  circle A14 centre (29.2853, 63.9396) radius 0.3175
  arc A15 (29.0948, 64.6116) -> (29.4758, 64.6116) centre (29.2853, 63.9396) ccw
  line L119 (29.0948, 64.9028) -> (29.0948, 64.6116)
  line L120 (29.0948, 64.9028) -> (25.8093, 64.9028)
  line L121 (22.9961, 65.2838) -> (29.0948, 65.2838)
  line L122 (29.4758, 64.6116) -> (29.4758, 67.2715)
  line L123 (29.0948, 67.2715) -> (29.0948, 65.2838)
  line L124 (22.9961, 65.2838) -> (31.6066, 70.2564)
  line L125 (31.9876, 66.1004) -> (31.9876, 65.8741)
  line L126 (31.9911, 70.2625) -> (31.9911, 66.4814)
  line L127 (20.9808, 64.9373) -> (31.7409, 71.0066)
  circle A16 centre (31.7971, 65.0383) radius 0.4127
  line L128 (31.75, 72.2052) -> (19.9413, 65.5444)
  line L129 (20.9808, 52.1009) -> (20.9808, 64.9373)
  line L130 (19.9413, 65.5444) -> (19.9413, 51.51)
  circle A17 centre (31.7313, 51.824) radius 0.4127
  line L131 (31.5408, 46.3613) -> (21.4951, 52.278)
  line L132 (19.9413, 51.51) -> (31.7966, 44.45)
  line L133 (31.8107, 45.6515) -> (20.9808, 52.1009)
  line L134 (31.5408, 49.8815) -> (26.3439, 52.8489)
  line L135 (26.3439, 52.4415) -> (31.5408, 49.4741)
  line L136 (31.5408, 51.0535) -> (31.5408, 49.8815)
  arc A18 (31.9218, 51.0535) -> (31.5408, 51.0535) centre (31.7313, 51.824) ccw
  circle A19 centre (41.0606, 62.1232) radius 0.381
  line L137 (40.8701, 59.3346) -> (39.5527, 59.3346)
  line L138 (39.4243, 58.9536) -> (40.8701, 58.9536)
  line L139 (37.7054, 52.5185) -> (37.7054, 53.0908)
  circle A20 centre (37.8959, 53.9267) radius 0.4763
  line L140 (38.7282, 53.737) -> (42.0481, 53.737)
  line L141 (38.0845, 53.0941) -> (38.0845, 52.3272)
  arc A21 (38.7317, 54.1172) -> (37.7054, 53.0908) centre (37.8959, 53.9267) ccw
  arc A22 (38.0845, 53.0941) -> (38.7282, 53.737) centre (37.8959, 53.9267) ccw
  line L142 (42.0481, 53.737) -> (42.0481, 52.1761)
  line L143 (43.5019, 51.0525) -> (43.5019, 65.3384)
  line L144 (42.4624, 64.7418) -> (42.4624, 51.6596)
  line L145 (41.2511, 61.3863) -> (41.2511, 54.1172)
  line L146 (39.4243, 58.9536) -> (38.6183, 59.7969)
  line L147 (39.5527, 59.3346) -> (38.9824, 59.9313)
  arc A23 (41.2511, 61.3863) -> (40.8701, 61.3863) centre (41.0606, 62.1232) ccw
  line L148 (38.3095, 61.5459) -> (38.3095, 62.5274)
  arc A24 (38.9824, 59.9313) -> (38.6905, 61.5459) centre (38.5, 60.6778) ccw
  line L149 (40.8701, 59.3346) -> (40.8701, 61.3863)
  line L150 (42.0481, 64.4224) -> (42.0481, 54.1172)
  line L151 (42.0481, 54.1172) -> (41.2511, 54.1172)
  line L152 (40.8701, 54.1172) -> (40.8701, 58.9536)
  line L153 (40.8701, 54.1172) -> (38.7317, 54.1172)
  arc A25 (38.3095, 61.5459) -> (38.6183, 59.7969) centre (38.5, 60.6778) ccw
  line L154 (43.5019, 65.3384) -> (31.75, 72.2052)
  line L155 (31.7409, 71.0066) -> (42.4624, 64.7418)
  line L156 (38.5023, 66.4814) -> (31.9911, 66.4814)
  line L157 (31.9876, 70.2646) -> (38.5023, 66.4814)
  line L158 (31.9911, 66.4814) -> (31.9911, 70.2625)
  line L159 (31.9911, 70.2625) -> (38.5023, 66.4814)
  line L160 (31.9911, 66.4814) -> (38.5023, 66.4814)
  line L161 (28.0615, 58.9484) -> (28.0615, 61.2883)
  line L162 (29.8151, 63.1194) -> (30.9581, 63.1194)
  line L163 (30.9581, 63.1194) -> (30.9581, 58.9484)
  line L164 (29.8151, 58.9484) -> (28.0615, 61.2883)
  line L165 (33.8556, 61.9764) -> (32.6087, 61.9764)
  line L166 (31.4657, 63.1194) -> (33.8556, 63.1194)
  line L167 (33.8556, 63.1194) -> (33.8556, 61.9764)
  line L168 (31.4657, 58.9484) -> (31.4657, 63.1194)
  line L169 (31.4657, 63.1194) -> (32.6087, 63.1194)
  line L170 (29.8151, 60.7795) -> (29.8151, 63.1194)
  line L171 (28.0615, 63.1194) -> (29.8151, 60.7795)
  line L172 (31.4657, 61.9764) -> (31.4657, 63.1194)
  line L173 (22.6601, 31.2964) -> (22.6651, 29.8066)
  line L174 (22.6665, 29.4256) -> (22.6651, 29.8066)
  line L175 (22.6507, 34.0285) -> (22.6587, 31.6774)
  line L176 (21.5243, 35.8431) -> (25.9921, 35.8584)
  line L177 (25.9908, 36.2394) -> (21.523, 36.2241)
  line L178 (22.2842, 29.8053) -> (21.5449, 29.8027)
  line L179 (21.5462, 29.4217) -> (22.2855, 29.4243)
  circle A26 centre (22.4578, 34.7329) radius 0.3493
  arc A27 (22.6507, 34.0285) -> (22.2697, 34.0272) centre (22.4578, 34.7329) ccw
  line L180 (22.2842, 29.8053) -> (22.2697, 34.0272)
  line L181 (21.523, 36.2241) -> (21.5243, 35.8431)
  line L182 (21.0767, 36.7309) -> (21.12, 24.0813)
  line L183 (19.9676, 23.5047) -> (19.9586, 37.4674)
  line L184 (21.5221, 36.4783) -> (21.5449, 29.8027)
  line L185 (26.9619, 31.6921) -> (22.6587, 31.6774)
  line L186 (22.6601, 31.2964) -> (26.9632, 31.3111)
  line L187 (26.9632, 31.3111) -> (26.9619, 31.6921)
  arc A28 (25.8644, 28.2691) -> (25.4834, 28.2678) centre (25.6715, 28.9736) ccw
  circle A29 centre (25.6715, 28.9736) radius 0.3493
  line L188 (31.8713, 16.6404) -> (19.9676, 23.5047)
  line L189 (21.12, 24.0813) -> (31.8964, 17.907)
  line L190 (23.0676, 23.4777) -> (31.6951, 18.5346)
  line L191 (29.165, 23.8796) -> (29.164, 24.1708)
  line L192 (29.1731, 21.5109) -> (29.1663, 23.4986)
  line L193 (29.1731, 21.5109) -> (29.174, 21.2473)
  line L194 (29.545, 24.1721) -> (29.5541, 21.5122)
  line L195 (29.5541, 21.5122) -> (31.6891, 20.289)
  line L196 (29.174, 21.2473) -> (31.6907, 19.8053)
  line L197 (31.6801, 22.9169) -> (31.6891, 20.289)
  line L198 (31.6907, 19.8053) -> (31.6951, 18.5346)
  line L199 (32.0796, 18.5298) -> (32.0667, 22.3109)
  line L200 (32.0618, 22.6919) -> (32.0611, 22.9182)
  circle A30 centre (31.8677, 23.7534) radius 0.4127
  arc A31 (32.0611, 22.9182) -> (31.6801, 22.9169) centre (31.8677, 23.7534) ccw
  circle A32 centre (41.1212, 26.7001) radius 0.381
  arc A33 (40.9282, 27.4363) -> (41.3092, 27.4376) centre (41.1212, 26.7001) ccw
  line L201 (40.9212, 29.488) -> (40.9282, 27.4363)
  circle A34 centre (38.5556, 28.1368) radius 0.508
  line L202 (40.9212, 29.488) -> (39.6037, 29.4835)
  arc A35 (38.7491, 27.2693) -> (39.0355, 28.8849) centre (38.5556, 28.1368) ccw
  line L203 (39.6037, 29.4835) -> (39.0355, 28.8849)
  line L204 (39.474, 29.8641) -> (40.9199, 29.869)
  line L205 (39.474, 29.8641) -> (38.6709, 29.0181)
  line L206 (42.1166, 24.4043) -> (42.0813, 34.7095)
  line L207 (42.562, 24.1393) -> (42.5183, 36.9086)
  line L208 (43.6866, 37.5937) -> (43.6957, 23.5059)
  line L209 (41.3092, 27.4376) -> (41.2843, 34.7068)
  line L210 (40.9033, 34.7055) -> (40.9199, 29.869)
  line L211 (38.7601, 35.0783) -> (42.08, 35.0897)
  line L212 (40.9033, 34.7055) -> (38.7649, 34.6981)
  line L213 (26.9772, 27.2181) -> (25.868, 27.2143)
  line L214 (25.8693, 26.8333) -> (26.9785, 26.8371)
  line L215 (25.868, 27.2143) -> (25.8644, 28.2691)
  line L216 (25.868, 27.2143) -> (25.8682, 27.1538)
  line L217 (22.6739, 27.2564) -> (22.6665, 29.4256)
  line L218 (22.2855, 29.4243) -> (22.2934, 27.1057)
  line L219 (25.4834, 28.2678) -> (25.4952, 24.8108)
  line L220 (22.6739, 27.2564) -> (25.4952, 24.8108)
  line L221 (21.5462, 29.4217) -> (21.5636, 24.3395)
  line L222 (25.8795, 23.8684) -> (25.8693, 26.8333)
  line L223 (25.4985, 23.8671) -> (22.4066, 23.8565)
  line L224 (21.5636, 24.3395) -> (22.4066, 23.8565)
  line L225 (22.2934, 27.1057) -> (25.4969, 24.3288)
  line L226 (25.9921, 35.8584) -> (26.0007, 33.3235)
  line L227 (26.3804, 33.7058) -> (26.3728, 35.924)
  line L228 (25.9885, 36.9013) -> (25.9908, 36.2394)
  line L229 (26.3714, 36.3314) -> (26.3695, 36.9026)
  line L230 (26.9563, 33.3268) -> (26.955, 33.7078)
  line L231 (26.955, 33.7078) -> (26.3804, 33.7058)
  line L232 (25.9994, 33.7045) -> (26.0007, 33.3235)
  line L233 (26.0007, 33.3235) -> (26.3817, 33.3248)
  line L234 (26.0007, 33.3235) -> (26.9563, 33.3268)
  line L235 (26.954, 34.0219) -> (26.9505, 35.0379)
  line L236 (25.4819, 28.6948) -> (25.482, 28.6802)
  line L237 (25.4969, 24.3288) -> (25.4985, 23.8671)
  line L238 (30.5693, 35.0503) -> (30.8814, 34.2954)
  line L239 (29.2143, 34.0297) -> (28.097, 34.0258)
  line L240 (29.4263, 35.0464) -> (30.5693, 35.0503)
  line L241 (29.4263, 35.0464) -> (30.8931, 30.8743)
  line L242 (26.9505, 35.0379) -> (26.9648, 30.8608)
  line L243 (29.2108, 35.0457) -> (29.2143, 34.0297)
  line L244 (28.1078, 30.8647) -> (28.097, 34.0258)
  circle A36 centre (31.7568, 36.9673) radius 0.4127
  line L245 (31.9366, 40.0825) -> (38.1116, 36.4859)
  line L246 (31.938, 39.6686) -> (37.7332, 36.2932)
  line L247 (30.8814, 34.2954) -> (32.1514, 34.2998)
  line L248 (32.4805, 35.0569) -> (32.1514, 34.2998)
  line L249 (33.9429, 35.0619) -> (35.9079, 35.0686)
  line L250 (31.081, 33.4233) -> (31.9594, 33.4263)
  line L251 (31.523, 32.3682) -> (31.081, 33.4233)
  line L252 (31.9594, 33.4263) -> (31.523, 32.3682)
  line L253 (35.0384, 34.1097) -> (35.6249, 34.1117)
  line L254 (35.041, 33.3599) -> (35.6356, 33.3619)
  circle A37 centre (37.9285, 34.8858) radius 0.4763
  arc A38 (37.7351, 35.7209) -> (38.7649, 34.6981) centre (37.9285, 34.8858) ccw
  arc A39 (36.3784, 32.8027) -> (35.9079, 35.0686) centre (35.9728, 33.9003) ccw
  line L255 (33.9054, 29.8503) -> (33.9093, 28.7073)
  line L256 (31.938, 39.6686) -> (31.9446, 37.7385)
  line L257 (35.0461, 31.8563) -> (35.4817, 31.8578)
  line L258 (32.4805, 35.0569) -> (33.6235, 35.0608)
  line L259 (35.0438, 32.5368) -> (35.4794, 32.5383)
  line L260 (35.0384, 34.1097) -> (35.041, 33.3599)
  arc A40 (35.6356, 33.3619) -> (35.6249, 34.1117) centre (35.597, 33.7363) ccw
  line L261 (35.0438, 32.5368) -> (35.0461, 31.8563)
  arc A41 (35.4817, 31.8578) -> (35.4794, 32.5383) centre (35.375, 32.1977) ccw
  arc A42 (35.9222, 30.8915) -> (36.3784, 32.8027) centre (35.6902, 31.9569) ccw
  line L262 (33.9572, 30.8847) -> (35.9222, 30.8915)
  line L263 (33.6235, 35.0608) -> (32.1631, 30.8786)
  line L264 (33.9429, 35.0619) -> (33.9572, 30.8847)
  line L265 (42.0813, 34.7095) -> (41.2843, 34.7068)
  line L266 (42.08, 35.0897) -> (42.0747, 36.6505)
  line L267 (26.9648, 30.8608) -> (28.1078, 30.8647)
  line L268 (28.1256, 25.6594) -> (26.9826, 25.6555)
  line L269 (26.9785, 26.8371) -> (26.9772, 27.2181)
  line L270 (26.9826, 25.6555) -> (26.9683, 29.8265)
  line L271 (26.9683, 29.8265) -> (28.1113, 29.8304)
  line L272 (28.1113, 29.8304) -> (28.1193, 27.4905)
  line L273 (28.1256, 25.6594) -> (29.8712, 28.0053)
  line L274 (29.8649, 29.8364) -> (28.1193, 27.4905)
  line L275 (29.8712, 28.0053) -> (29.8792, 25.6654)
  line L276 (31.0079, 29.8403) -> (29.8649, 29.8364)
  line L277 (31.0222, 25.6693) -> (31.0079, 29.8403)
  circle A43 centre (29.3522, 24.8434) radius 0.3175
  line L278 (29.8792, 25.6654) -> (31.0222, 25.6693)
  arc A44 (29.545, 24.1721) -> (29.164, 24.1708) centre (29.3522, 24.8434) ccw
  line L279 (38.3728, 25.9055) -> (38.3837, 22.7135)
  line L280 (38.7647, 22.7148) -> (38.7491, 27.2693)
  line L281 (38.3681, 27.268) -> (38.3715, 26.2865)
  circle A45 centre (26.1761, 37.735) radius 0.4762
  arc A46 (26.3695, 36.9026) -> (25.9885, 36.9013) centre (26.1761, 37.735) ccw
  line L282 (28.0935, 35.0418) -> (26.9505, 35.0379)
  line L283 (26.9505, 35.0379) -> (29.2108, 35.0457)
  line L284 (31.5582, 39.3166) -> (31.5476, 42.4293)
  line L285 (31.5596, 38.9092) -> (26.3728, 35.924)
  line L286 (26.3714, 36.3314) -> (31.5582, 39.3166)
  line L287 (31.5476, 42.4293) -> (21.5221, 36.4783)
  line L288 (31.7603, 43.0725) -> (21.0767, 36.7309)
  line L289 (19.9586, 37.4674) -> (31.7966, 44.45)
  line L290 (31.9286, 42.4307) -> (31.9366, 40.0825)
  line L291 (31.9286, 42.4307) -> (31.9285, 42.4639)
  line L292 (31.7966, 44.45) -> (43.6866, 37.5937)
  line L293 (42.5183, 36.9086) -> (31.7603, 43.0725)
  line L294 (42.0747, 36.6505) -> (31.9285, 42.4639)
  line L295 (31.5636, 37.7372) -> (31.5596, 38.9092)
  arc A47 (31.5636, 37.7372) -> (31.9446, 37.7385) centre (31.7568, 36.9673) ccw
  line L296 (38.1142, 35.719) -> (38.1116, 36.4859)
  arc A48 (38.7601, 35.0783) -> (38.1142, 35.719) centre (37.9285, 34.8858) ccw
  line L297 (37.7332, 36.2932) -> (37.7351, 35.7209)
  line L298 (38.3728, 25.9055) -> (37.1595, 25.9014)
  line L299 (37.1582, 26.2824) -> (38.3715, 26.2865)
  line L300 (37.1595, 25.9014) -> (37.1582, 26.2824)
  line L301 (36.3108, 29.8585) -> (35.1678, 29.8546)
  line L302 (34.347, 26.7047) -> (35.1786, 26.7075)
  line L303 (35.1678, 29.8546) -> (35.1786, 26.7075)
  line L304 (35.1786, 26.7075) -> (35.2746, 26.7079)
  line L305 (36.3215, 26.7115) -> (36.3108, 29.8585)
  line L306 (36.3215, 26.7115) -> (37.1567, 26.7143)
  line L307 (34.3505, 25.6887) -> (34.347, 26.7047)
  line L308 (37.1602, 25.6983) -> (34.3505, 25.6887)
  line L309 (37.1567, 26.7143) -> (37.1602, 25.6983)
  arc A49 (38.6709, 29.0181) -> (38.3681, 27.268) centre (38.5556, 28.1368) ccw
  line L310 (29.165, 23.8796) -> (25.8795, 23.8684)
  line L311 (23.0676, 23.4777) -> (29.1663, 23.4986)
  line L312 (30.8931, 30.8743) -> (32.1631, 30.8786)
  line L313 (33.9093, 28.7073) -> (32.6624, 28.703)
  line L314 (32.6638, 28.2849) -> (32.6624, 28.703)
  line L315 (33.9107, 28.2892) -> (32.6638, 28.2849)
  line L316 (33.9142, 27.2732) -> (33.9107, 28.2892)
  line L317 (32.6585, 29.846) -> (31.5155, 29.8421)
  line L318 (31.5155, 29.8421) -> (33.9054, 29.8503)
  line L319 (31.5194, 28.6991) -> (31.5155, 29.8421)
  line L320 (32.6673, 27.2689) -> (33.9142, 27.2732)
  line L321 (32.6688, 26.818) -> (32.6673, 27.2689)
  line L322 (33.9158, 26.8222) -> (32.6688, 26.818)
  line L323 (31.5155, 29.8421) -> (31.5298, 25.6711)
  line L324 (33.9197, 25.6792) -> (33.9158, 26.8222)
  line L325 (31.5298, 25.6711) -> (33.9197, 25.6792)
  line L326 (31.5298, 25.6711) -> (32.6728, 25.675)
  line L327 (31.5258, 26.8141) -> (31.5298, 25.6711)
  line L328 (31.5208, 28.281) -> (31.5243, 27.265)
  line L329 (39.2326, 22.7164) -> (42.1166, 24.4043)
  line L330 (38.7647, 22.7148) -> (39.2326, 22.7164)
  line L331 (35.6693, 22.7042) -> (38.3837, 22.7135)
  line L332 (35.2848, 23.7486) -> (35.2883, 22.7029)
  circle A50 centre (35.4727, 24.4871) radius 0.3175
  arc A51 (35.6658, 23.7499) -> (35.2848, 23.7486) centre (35.4727, 24.4871) ccw
  line L333 (32.0618, 22.6919) -> (35.2883, 22.7029)
  line L334 (35.6693, 22.7042) -> (35.6658, 23.7499)
  line L335 (38.5779, 22.3332) -> (32.0667, 22.3109)
  line L336 (32.0667, 22.3109) -> (38.5779, 22.3332)
  line L337 (31.8964, 17.907) -> (42.562, 24.1393)
  line L338 (43.6957, 23.5059) -> (31.8713, 16.6404)
  line L339 (32.0796, 18.5298) -> (38.5779, 22.3332)
  line L340 (32.0761, 18.5277) -> (38.5779, 22.3332)
  line L341 (32.0667, 22.3109) -> (32.0796, 18.5298)
  line L342 (31.75, 80.4139) -> (44.6823, 72.8573)
  line L343 (44.6823, 72.8573) -> (54.0323, 76.3351)
  line L344 (54.0323, 76.3351) -> (63.5, 70.8029)
  line L345 (31.75, 72.2052) -> (31.75, 88.9) construction
  line L346 (31.75, 80.4139) -> (18.8177, 72.8573)
  line L347 (18.8177, 72.8573) -> (9.4677, 76.3351)
  line L348 (9.4677, 76.3351) -> (0, 70.8029)
  line L349 (29.1432, 44.45) -> (63.5, 44.45) construction
  line L350 (9.4677, 12.5649) -> (0, 18.0971)
  line L351 (18.8177, 16.0427) -> (9.4677, 12.5649)
  line L352 (31.75, 8.4861) -> (18.8177, 16.0427)
  line L353 (31.75, 8.4861) -> (44.6823, 16.0427)
  line L354 (44.6823, 16.0427) -> (54.0323, 12.5649)
  line L355 (54.0323, 12.5649) -> (63.5, 18.0971)
  line L356 (0, 51.1737) -> (17.8526, 51.1737)
  line L357 (17.8526, 51.1737) -> (29.1432, 44.45)
  line L358 (17.8526, 37.7263) -> (29.1432, 44.45)
  line L359 (0, 37.7263) -> (17.8526, 37.7263)
  line L360 (63.5, 51.1737) -> (45.6474, 51.1737)
  line L361 (45.6474, 51.1737) -> (34.3568, 44.45)
  line L362 (45.6474, 37.7263) -> (34.3568, 44.45)
  line L363 (63.5, 37.7263) -> (45.6474, 37.7263)
  point P0 (31.7785, 58.3278)
  point P1 (31.8262, 30.4638)
  point P2 (-146.0528, 86.9255)
  point P3 (-156.4796, 93.0964)
  point P4 (-151.6308, 96.0123)
  point P5 (-151.0562, 96.0123)
  point P6 (-151.0562, 97.647)
  point P7 (-145.9836, 110.8267)
  point P8 (-151.0562, 98.028)
  point P9 (-149.9132, 94.3011)
  point P10 (-151.0562, 95.3171)
  point P11 (-151.0562, 95.6313)
  point P12 (-140.8785, 103.0916)
  point P13 (-140.8785, 103.4726)
  point P14 (-151.0562, 102.502)
  point P15 (-151.0562, 102.121)
  point P16 (-145.366, 99.5126)
  point P17 (-146.509, 100.6556)
  point P18 (-146.509, 101.0737)
  point P19 (-146.0461, 82.9948)
  point P20 (-156.4517, 76.7883)
  point P21 (-151.0128, 72.2563)
  point P22 (-151.0183, 73.8909)
  point P23 (-151.593, 73.889)
  point P24 (-150.9974, 67.7823)
  point P25 (-150.9961, 67.4013)
  point P26 (-140.8152, 66.4656)
  point P27 (-140.8165, 66.8466)
  point P28 (-151.0196, 74.2719)
  point P29 (-151.0207, 74.5861)
  point P30 (-149.8812, 75.606)
  point P31 (-151.0114, 71.8753)
  point P32 (-146.4553, 69.2633)
  point P33 (-145.3162, 70.4102)
  point P34 (-114.4747, 58.6613)
  point P35 (-177.9747, 58.6613)
  point P36 (-177.9747, 111.3671)
  dimension "d17" = 63.5
  dimension "d18" = 88.9
  constraints: 728 end point, 89 parallel, 64 point on circle, 50 centre point, 37 horizontal, 22 point on line, 21 perpendicular, 20 coincident, 17 symmetric about line, 5 vertical, 4 collinear, 2 midpoint, 11 other
  measures "d17" distance of L2.end L1.end
  measures "d18" distance of L1.end L0.end